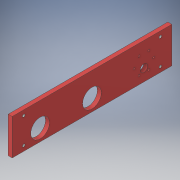
# Autodesk Inventor part: DriveRail
Saved by Autodesk Inventor 2018 (Build 220112000, 112)
## iProperties
Created: 2017-12-20
Part Number: DriveRail
Material: Generic
Document SubType Name: Modeling
Designer: jklei
Density: 1 g/cm^3
Appearance: Default
Author: jklei
Autodesk Inventor part; units mm, degrees
ref_plane "YZ Plane" through (0, 0, 0) normal (1, 0, 0) x (0, 1, 0)
ref_plane "XZ Plane" through (0, 0, 0) normal (0, 1, 0) x (-1, 0, 0)
ref_plane "XY Plane" through (0, 0, 0) normal (0, 0, 1) x (1, 0, 0)
sketch "Sketch1" plane through (0, 0, 0) normal (1, 0, 0) x (0, 1, 0)
  line L0 (0, 0) -> (57.15, 0)
  line L1 (57.15, 0) -> (57.15, -254)
  line L2 (57.15, -254) -> (0, -254)
  line L3 (0, -254) -> (0, 0)
  dimension "d0" = 57.15
  dimension "d1" = 254
  constraints: 8 end point, 2 parallel, 1 horizontal, 1 perpendicular
  measures "d0" distance of L1.end L2.end
  measures "d1" distance of L0.end L1.end
extrude "Extrusion1" add sketch "Sketch1" along normal blind 6.35
sketch "Sketch2" plane through (6.35, 0, 0) normal (1, 0, 0) x (0, 0, -1)
  line L0 (254, 57.15) -> (0, 57.15) projected
  circle A0 centre (209.55, 19.05) radius 5.9944
  line L1 (209.55, 19.05) -> (209.55, 26.0604)
  circle A1 centre (209.55, 26.0604) radius 15.494
  circle A2 centre (225.044, 26.0604) radius 1.4986
  circle A3 centre (217.297, 39.4786) radius 1.4986
  circle A4 centre (201.803, 39.4786) radius 1.4986
  circle A5 centre (194.056, 26.0604) radius 1.4986
  circle A6 centre (201.803, 12.6422) radius 1.4986
  circle A7 centre (217.297, 12.6422) radius 1.4986
  line L2 (209.55, 13.0556) -> (0, 13.0556)
  line L3 (0, 57.15) -> (0, 0) projected
  line L4 (0, 0) -> (254, 0) projected
  dimension "d7" = 11.9888
  dimension "d9" = 7.0104
  dimension "d10" = 30.988
  dimension "d11" = 2.9972
  dimension "d14" = 360
  dimension "d28" = 209.55
  dimension "d49" = 13.0556
  constraints: 7 centre point, 4 end point, 1 coincident, 1 horizontal, 1 point on line, 1 vertical alignment, 15 other
  measures "d9" distance of L1.start L1.end
  measures "d10" diameter of A1
  measures "d11" diameter of A2
  measures "d28" distance of L2.start L2.end
  measures "d49" distance between parallel lines of L4 L2
extrude "Extrusion2" cut sketch "Sketch2" against normal through all contours A0 | A1 A2 | A1 A2 | A3 A1 | A1 A3 | A7 A1 | A1 A7 | A4 A1 | A1 A4 | A6 L2 A1 | A1 L2 A6 | L2 A6 A1 | A1 A6 L2 | A5 A1 | A1 A5
sketch "Sketch3" plane through (6.35, 0, 0) normal (1, 0, 0) x (0, 0, -1)
  circle A0 centre (209.55, 19.05) radius 5.9944 projected
  circle A1 centre (201.803, 12.6422) radius 1.4986 projected
  circle A2 centre (201.803, 39.4786) radius 1.4986 projected
  circle A3 centre (225.044, 26.0604) radius 1.4986 projected
  circle A4 centre (217.297, 39.4786) radius 1.4986 projected
  circle A5 centre (194.056, 26.0604) radius 1.4986 projected
  circle A6 centre (217.297, 12.6422) radius 1.4986 projected
  line L0 (0, 57.15) -> (0, 0) projected
  line L1 (0, 0) -> (254, 0) projected
  line L2 (254, 0) -> (254, 57.15) projected
  line L3 (254, 57.15) -> (0, 57.15) projected
  line L4 (209.55, 19.05) -> (127, 19.05)
  circle A7 centre (127, 19.05) radius 14.9225
  circle A8 centre (127, 19.05) radius 36.5125
  line L5 (127, 19.05) -> (44.45, 19.05)
  circle A9 centre (44.45, 19.05) radius 14.9225
  dimension "d18" = 82.55
  dimension "d19" = 29.845
  dimension "d27" = 73.025
  dimension "d29" = 82.55
  dimension "d30" = 29.845
  constraints: 4 end point, 3 centre point, 3 coincident, 2 horizontal
  measures "d18" distance of L4.start L4.end
  measures "d19" diameter of A7
  measures "d27" diameter of A8
  measures "d29" distance of L5.start L5.end
  measures "d30" diameter of A9
extrude "Extrusion3" cut sketch "Sketch3" against normal through all contours L5 L4 A7 | A7 L4 L5 | A9
sketch "Sketch4" plane through (6.35, 0, 0) normal (1, 0, 0) x (0, 0, -1)
  line L0 (0, 57.15) -> (0, 0) projected
  line L1 (254, 0) -> (254, 57.15) projected
  line L2 (0, 57.15) -> (6.35, 57.15)
  line L3 (6.35, 57.15) -> (18.35, 57.15)
  line L4 (18.35, 57.15) -> (18.35, 49.15)
  circle A0 centre (18.35, 49.15) radius 2.1
  line L5 (6.35, 0) -> (18.35, 0)
  line L6 (18.35, 0) -> (18.35, 8)
  circle A1 centre (18.35, 8) radius 2.1
  line L7 (254, 57.15) -> (247.65, 57.15)
  line L8 (247.65, 57.15) -> (235.65, 57.15)
  line L9 (247.65, 0) -> (235.65, 0)
  circle A2 centre (235.65, 49.15) radius 2.1
  circle A3 centre (235.65, 8) radius 2.1
  line L10 (254, 57.15) -> (0, 57.15) projected
  dimension "d31" = 6.35
  dimension "d32" = 12
  dimension "d33" = 8
  dimension "d34" = 4.2
  dimension "d35" = 12
  dimension "d36" = 8
  dimension "d37" = 4.2
  dimension "d38" = 6.35
  dimension "d39" = 12
  dimension "d41" = 12
  dimension "d43" = 4.2
  dimension "d44" = 4.2
  dimension "d45" = 6.35
  dimension "d46" = 6.35
  constraints: 16 end point, 4 centre point, 2 coincident, 2 perpendicular
  measures "d31" distance of L0.start L2.end
  measures "d32" distance of L2.end L3.end
  measures "d33" distance of L3.end L4.end
  measures "d34" diameter of A0
  measures "d35" distance of L5.start L5.end
  measures "d36" distance of L5.end L6.end
  measures "d37" diameter of A1
  measures "d38" distance of L1.end L7.end
  measures "d39" distance of L7.end L8.end
  measures "d41" distance of L9.start L9.end
  measures "d43" diameter of A2
  measures "d44" diameter of A3
  measures "d45" distance of L1.start L9.start
  measures "d46" distance of point (0, 0) L5.start
extrude "Extrusion4" cut sketch "Sketch4" against normal through all
body "Solid1"
